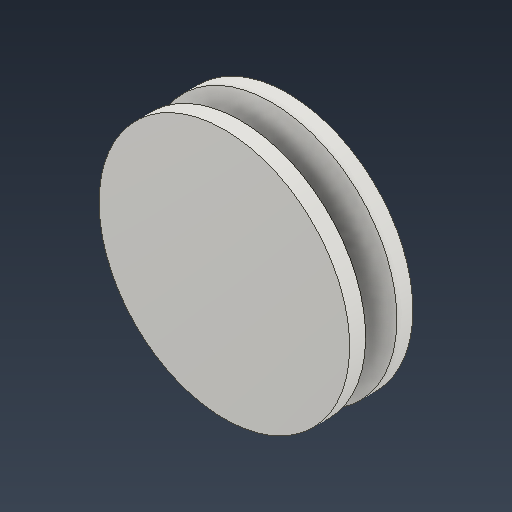
# Autodesk Inventor part: Шкив желобчатый2
Saved by Autodesk Inventor 2026 (Build 300175000, 175)
## iProperties
Created: 2026-01-10
Part Number: Шкив желобчатый2
Material: Steel
Document SubType Name: Modeling
Designer: GameHD
Density: 1 g/cm^3
Appearance: Steel
CustomPartVersion: 1
Author: GameHD
Autodesk Inventor part; units mm, degrees
ref_plane "YZ Plane" through (0, 0, 0) normal (1, 0, 0) x (0, 1, 0)
ref_plane "XZ Plane" through (0, 0, 0) normal (0, 1, 0) x (-1, 0, 0)
sketch "Основной эскиз" plane through (0, 0, 0) normal (1, 0, 0) x (0, 1, 0)
  line L0 (0, 10) -> (19.8, 10)
  line L1 (19.8, 10) -> (19.8, 7.4728)
  line L2 (19.8, 7.4728) -> (13.8, 5.7523)
  line L3 (13.8, 5.7523) -> (13.8, 4.2477)
  line L4 (13.8, 4.2477) -> (19.8, 2.5272)
  line L5 (19.8, 2.5272) -> (19.8, 0)
  line L6 (19.8, 0) -> (0, 0)
  line L7 (18.5, 7.1) -> (18.5, 2.9) construction
  line L8 (13.8, 5) -> (18.5, 5) construction
  line L9 (19.8, 7.4728) -> (19.8, 2.5272)
  line L10 (0, -2) -> (0, 12) projected
  line L11 (0, 0) -> (0, 10)
  dimension "d0" = 4.2
  dimension "d1" = 32
  dimension "d2" = 1.3
  dimension "d6" = 10
  dimension "d21" = 37
  dimension "d25" = 6
  dimension "d27" = 5
  constraints: 22 end point, 5 perpendicular, 2 collinear, 2 midpoint, 2 point on line, 1 parallel
  measures "d0" distance of L7.start L7.end
  measures "d1" angle of L2 L4
  measures "d2" distance between parallel lines of L1 L7
  measures "d6" distance between parallel lines of L6 L0
  measures "d21" diameter of L7 L10
  measures "d25" distance between parallel lines of L3 L9
  measures "d27" distance between parallel lines of L6 L8
ref_plane "Плоскость ремня" through (0, 13.8, 5) normal (0, 0, 1) x (1, 0, 0)
revolve "Тело" add sketch "Основной эскиз" angle 360 about axis through (0, 0, -10) along (0, 0, 1)
revolve "Канавка" cut sketch "Основной эскиз" angle 360 about axis through (0, 0, -10) along (0, 0, 1) contours L9 L4 L3 L2
fillet "Сопряжение снаружи" [suppressed]
fillet "Сопряжение изнутри" [suppressed]
pattern_of_one "Образец канавки"
equation "\"d0\" = da_Bw"
equation "\"d1\" = da_Alfa"
equation "\"d2\" = da_c"
equation "\"d21\" = da_Dw"
equation "\"d25\" = da_Hd"
equation "\"d27\" = da_Se"
equation "\"da_r1\" = 0"
equation "\"da_r2\" = 0"
equation "\"d18\" = da_Sg"
equation "\"d5\" = da_Se"
equation "\"da_Bw\" = 4.2"
equation "\"da_Alfa\" = 32deg"
equation "\"da_c\" = 1.3"
equation "\"da_Dw\" = 37"
equation "\"da_Hd\" = 6"
equation "\"da_Se\" = 5"
equation "\"da_Sg\" = 6"
body "Solid1"
